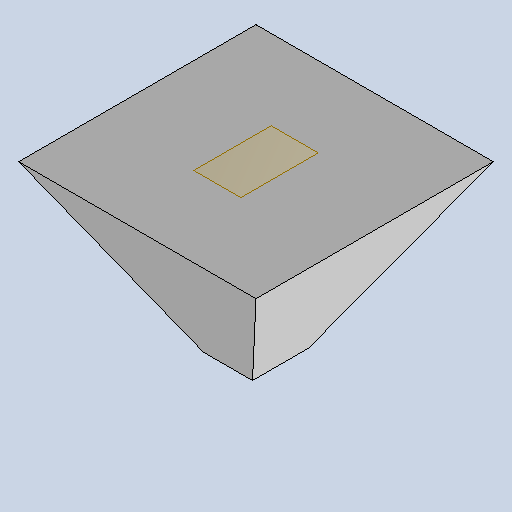
# Autodesk Inventor part: NDM-VOS dummy2
Saved by Autodesk Inventor 2025 (Build 290162010, 162A)
## iProperties
Created: 2024-07-24
Part Number: NDM-VOS dummy2
Material: Water
Document SubType Name: Modeling
Designer: admin
Mass: 1.00163e+06 g
Surface Area: 67468.3 cm^2
Volume: 1.00333e+06 cm^3
Density: 0.9983 g/cm^3
Appearance: Default
Author: admin
Autodesk Inventor part; units mm, degrees
ref_plane "YZ Plane" through (0, 0, 0) normal (1, 0, 0) x (0, 1, 0)
ref_plane "XZ Plane" through (0, 0, 0) normal (0, 1, 0) x (-1, 0, 0)
sketch "Sketch2" plane through (0, 0, 0) normal (0, 0, 1) x (1, 0, 0)
  line L0 (175, -200) -> (-175, -200)
  line L1 (-175, -200) -> (-175, 200)
  line L2 (-175, 200) -> (175, 200)
  line L3 (175, 200) -> (175, -200)
  line L4 (175, -200) -> (-175, 200) construction
  line L5 (-175, -200) -> (175, 200) construction
  point P0 (0, 0)
  point P1 (0, 0)
  dimension "d9" = 400
  dimension "d16" = 350
  constraints: 12 end point, 2 coincident, 2 midpoint, 2 parallel, 1 horizontal, 1 perpendicular
  measures "d9" distance of L0.end L1.end
  measures "d16" distance of L0.start L0.end
ref_plane "Work Plane1" through (0, 0, 1170) normal (0, 0, 1) x (1, 0, 0)
sketch "Sketch3" plane through (0, 0, 1170) normal (0, 0, 1) x (1, 0, 0)
  line L0 (850, 850) -> (-850, 850)
  line L1 (-850, 850) -> (-850, -850)
  line L2 (-850, -850) -> (850, -850)
  line L3 (850, -850) -> (850, 850)
  line L4 (850, 850) -> (-850, -850) construction
  line L5 (-850, 850) -> (850, -850) construction
  point P0 (0, 0)
  point P1 (0, 0)
  dimension "d11" = 1700
  dimension "d17" = 1700
  constraints: 12 end point, 2 midpoint, 2 parallel, 1 coincident, 1 horizontal, 1 perpendicular
  measures "d11" distance of L0.end L1.end
  measures "d17" distance of L1.end L2.end
loft "Loft1" add profiles "Sketch3", "Sketch2"
equation "\"d9\" = Конус_дно_длина"
equation "\"d16\" = Конус_дно_ширина"
equation "\"d11\" = Конус_Базовая_длина"
equation "\"d17\" = Конус_Базовая_ширина"
equation "\"Конус_дно_длина\" = 400"
equation "\"Конус_дно_ширина\" = 350"
equation "\"Конус_Базовая_длина\" = 1700"
equation "\"Конус_Базовая_ширина\" = 1700"
body "Solid2"
